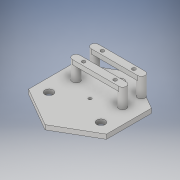
# Autodesk Inventor part: 80_20_Connector_Bot
Saved by Autodesk Inventor 2019 (Build 230136000, 136)
## iProperties
Created: 2019-08-10
Part Number: 80_20_Connector_Bot
Material: Generic
Document SubType Name: Modeling
Designer: Jorian Brusind
Density: 1 g/cm^3
Appearance: Default
Author: Jorian Brusind
Autodesk Inventor part; units mm, degrees
ref_plane "YZ Plane" through (0, 0, 0) normal (1, 0, 0) x (0, 1, 0)
ref_plane "XZ Plane" through (0, 0, 0) normal (0, 1, 0) x (-1, 0, 0)
ref_plane "XY Plane" through (0, 0, 0) normal (0, 0, 1) x (1, 0, 0)
sketch "Sketch1" plane through (0, 0, 0) normal (0, 1, 0) x (-1, 0, 0)
  line L0 (0, 0) -> (0, -30)
  circle A0 centre (0, 0) radius 30
  line L1 (0, -30) -> (-25.9808, -15)
  line L2 (0, -30) -> (30, -30) construction
  line L3 (-25.9808, -15) -> (-25.9808, 15)
  line L4 (-25.9808, -15) -> (4.0192, -15) construction
  line L5 (-25.9808, 15) -> (0, 30)
  line L6 (0, 30) -> (25.9808, 15)
  line L7 (25.9808, 15) -> (25.9808, -15)
  line L8 (0, -30) -> (25.9808, -15)
  dimension "d0" = 30
  dimension "d1" = 150
  dimension "d3" = 30
  dimension "d4" = 90
  dimension "d5" = 30
  dimension "d6" = 120
  dimension "d7" = 25.9808
  constraints: 18 end point, 3 point on circle, 2 equal length, 2 horizontal, 2 parallel, 2 vertical, 1 centre point, 1 coincident
  measures "d0" distance of L0.start L0.end
  measures "d1" angle of L2 L1
  measures "d3" distance of L1.end L3.end
  measures "d4" angle of L4 L3
  measures "d5" distance of L3.end L5.end
  measures "d6" angle of L3 L5
  measures "d7" horizontal distance of L0.end L1.end
extrude "Extrusion1" add sketch "Sketch1" along normal blind 3 contours L7 L8 L1 L3 L5 L6
sketch "Sketch2" plane through (0, 3, 0) normal (0, 1, 0) x (1, 0, 0)
  line L0 (0, 0) -> (0, 20)
  circle A0 centre (0, 20) radius 2.75
  line L1 (0, 0) -> (17.3205, -10)
  line L2 (0, 0) -> (20, 0) construction
  line L3 (0, 0) -> (-17.3205, -10)
  line L4 (0, 0) -> (20, 0) construction
  circle A1 centre (-17.3205, -10) radius 2.75
  circle A2 centre (17.3205, -10) radius 2.75
  dimension "d10" = 20
  dimension "d11" = 5.5
  dimension "d12" = 20
  dimension "d13" = 30
  dimension "d14" = 20
  dimension "d15" = 150
  dimension "d16" = 5.5
  dimension "d17" = 5.5
  constraints: 10 end point, 3 centre point, 3 coincident, 2 equal length, 2 horizontal, 1 vertical
  measures "d10" distance of L0.start L0.end
  measures "d11" diameter of A0
  measures "d12" distance of L0.start L1.end
  measures "d13" angle of L1 L2
  measures "d14" distance of L0.start L3.end
  measures "d15" angle of L3 L4
  measures "d16" diameter of A1
  measures "d17" diameter of A2
extrude "Extrusion2" cut sketch "Sketch2" against normal blind 10
sketch "Sketch3" plane through (0, 3, 0) normal (0, 1, 0) x (1, 0, 0)
  line L0 (0, 0) -> (0, 12.5)
  line L1 (10.5, 6.25) -> (-10.5, 6.25)
  line L2 (-10.5, 6.25) -> (-10.5, 18.75)
  line L3 (-10.5, 18.75) -> (10.5, 18.75)
  line L4 (10.5, 18.75) -> (10.5, 6.25)
  line L5 (10.5, 6.25) -> (-10.5, 18.75) construction
  line L6 (-10.5, 6.25) -> (10.5, 18.75) construction
  line L7 (-10.5, 18.75) -> (-15.5, 18.75)
  line L8 (-10.5, 6.25) -> (-15.5, 6.25)
  line L9 (10.5, 18.75) -> (15.5, 18.75)
  line L10 (10.5, 18.75) -> (15.5, 18.75) construction
  line L11 (10.5, 6.25) -> (15.5, 6.25)
  circle A0 centre (-15.5, 18.75) radius 2.5
  circle A1 centre (-15.5, 6.25) radius 2.5
  circle A2 centre (15.5, 18.75) radius 2.5
  circle A3 centre (15.5, 6.25) radius 2.5
  dimension "d20" = 12.5
  dimension "d21" = 21
  dimension "d22" = 12.5
  dimension "d29" = 5
  dimension "d30" = 5
  dimension "d31" = 5
  dimension "d32" = 0
  dimension "d33" = 5
  dimension "d34" = 5
  dimension "d35" = 5
  dimension "d36" = 5
  dimension "d37" = 5
  constraints: 24 end point, 6 horizontal, 4 centre point, 4 coincident, 2 midpoint, 2 parallel, 1 collinear, 1 perpendicular, 1 vertical
  measures "d20" distance of L0.start L0.end
  measures "d21" distance of L2.end L3.end
  measures "d22" distance of L1.end L2.end
  measures "d29" distance of L2.end L7.end
  measures "d30" distance of L1.end L8.end
  measures "d31" distance of L3.end L9.end
  measures "d32" distance between parallel lines of L9 L10
  measures "d33" distance of L1.start L11.end
  measures "d34" diameter of A0
  measures "d35" diameter of A1
  measures "d36" diameter of A2
  measures "d37" diameter of A3
extrude "Extrusion4" add sketch "Sketch3" along normal blind 10 contours A0 | A1 | A2 | A3
sketch "Sketch4" plane through (-15.5, 13, -18.75) normal (0, 1, 0) x (1, 0, 0)
  circle A0 centre (0, 0) radius 2.5 projected
  line L0 (0, 2.5) -> (31, 2.5)
  line L1 (31, 2.5) -> (31, -2.5)
  line L2 (31, -2.5) -> (0, -2.5)
  line L3 (0, -2.5) -> (0, 2.5)
  circle A1 centre (0, -12.5) radius 2.5 projected
  line L4 (0, -10) -> (31, -10)
  line L5 (31, -10) -> (31, -15)
  line L6 (31, -15) -> (0, -15)
  line L7 (0, -15) -> (0, -10)
  circle A2 centre (31, -12.5) radius 2.5 projected
  circle A3 centre (31, 0) radius 2.5 projected
  point P0 (15.5, -18.75)
  dimension "d40" = 31
  dimension "d41" = 5
  dimension "d42" = 2.5
  dimension "d43" = 31
  dimension "d44" = 5
  dimension "d49" = 2.5
  constraints: 16 end point, 4 parallel, 2 horizontal, 2 perpendicular, 2 vertical alignment, 2 other
  measures "d40" distance of L1.end L2.end
  measures "d41" distance of L0.end L1.end
  measures "d43" distance of L5.end L6.end
  measures "d44" distance of L4.end L5.end
extrude "Extrusion5" add sketch "Sketch4" along normal blind 3
sketch "Sketch5" plane through (-15.5, 16, -18.75) normal (0, 1, 0) x (1, 0, 0)
  circle A0 centre (0, 0) radius 2.5 projected
  line L0 (0, 0) -> (5, 0)
  arc A1 (31, -2.5) -> (31, 2.5) centre (31, 0) ccw projected
  line L1 (31, 0) -> (26, 0)
  circle A2 centre (0, -12.5) radius 2.5 projected
  line L2 (0, -12.5) -> (5, -12.5)
  circle A3 centre (31, -12.5) radius 2.5 projected
  line L3 (31, -12.5) -> (26, -12.5)
  circle A4 centre (5, 0) radius 1.15
  circle A5 centre (26, 0) radius 1.15
  circle A6 centre (5, -12.5) radius 1.15
  circle A7 centre (26, -12.5) radius 1.15
  point P0 (15.5, -18.75)
  dimension "d52" = 5
  dimension "d53" = 5
  dimension "d54" = 5
  dimension "d55" = 5
  dimension "d56" = 2.3
  dimension "d57" = 2.3
  dimension "d58" = 2.3
  dimension "d59" = 2.3
  constraints: 8 end point, 4 centre point, 4 coincident, 4 horizontal
  measures "d52" distance of L0.start L0.end
  measures "d53" distance of L1.start L1.end
  measures "d54" distance of L2.start L2.end
  measures "d55" distance of L3.start L3.end
  measures "d56" diameter of A4
  measures "d57" diameter of A5
  measures "d58" diameter of A6
  measures "d59" diameter of A7
extrude "Extrusion6" cut sketch "Sketch5" against normal blind 3 contours A4 | A5 | A6 | A7
sketch "Sketch6" plane through (0, 3, 0) normal (0, 1, 0) x (1, 0, 0)
  circle A0 centre (0, 0) radius 1
  dimension "d62" = 2
  constraints: 1 centre point, 1 coincident
  measures "d62" diameter of A0
extrude "Extrusion7" cut sketch "Sketch6" against normal blind 10
body "Solid1"
